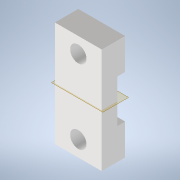
# Autodesk Inventor part: Encoder_Cable_Clamp
Saved by Autodesk Inventor 2022 (Build 260153000, 153)
## iProperties
Created: 2024-05-02
Part Number: Encoder_Cable_Clamp
Material: Generic
Document SubType Name: Modeling
Designer: Gotham City
Density: 1 g/cm^3
Appearance: Default
Author: Gotham City
Autodesk Inventor part; units mm, degrees
ref_plane "YZ Plane" through (0, 0, 0) normal (1, 0, 0) x (0, 1, 0)
ref_plane "XZ Plane" through (0, 0, 0) normal (0, 1, 0) x (-1, 0, 0)
ref_plane "XY Plane" through (0, 0, 0) normal (0, 0, 1) x (1, 0, 0)
sketch "Sketch1" plane through (0, 0, 0) normal (1, 0, 0) x (0, 1, 0)
  line L0 (-0.5, 0) -> (0.55, 0) projected
  line L1 (3.0679, 1.692) -> (-10.4321, 1.692)
  line L2 (-10.4321, 1.692) -> (-10.4321, 4.692)
  line L3 (-10.4321, 4.692) -> (3.0679, 4.692)
  line L4 (3.0679, 4.692) -> (3.0679, 1.692)
  line L5 (-0.9321, 1.692) -> (-6.4321, 1.692)
  line L6 (-6.4321, 1.692) -> (-6.4321, 2.692)
  line L7 (-6.4321, 2.692) -> (-0.9321, 2.692)
  line L8 (-0.9321, 2.692) -> (-0.9321, 1.692)
  line L9 (-3.6821, 1.692) -> (-3.6821, 4.692) construction
  line L10 (1.0679, 4.692) -> (1.0679, 1.692) construction
  line L11 (-0.5, 0) -> (0.55, 0) construction
  point P0 (0, 0)
  dimension "d0" = 5.5
  dimension "d1" = 4
  dimension "d2" = 2
  dimension "d3" = 1
  dimension "d4" = 2
  constraints: 20 end point, 4 parallel, 4 perpendicular, 3 point on line, 2 horizontal, 2 midpoint, 1 other
  measures "d0" distance of L6.end L7.end
  measures "d1" distance between parallel lines of L4 L8
  measures "d2" distance between parallel lines of L3 L7
  measures "d3" distance between parallel lines of L1 L7
  measures "d4" distance between parallel lines of L8 L10
extrude "Extrusion1" add sketch "Sketch1" along normal blind 6 contours L1 L8 L7 L6 L2 L3 L4
sketch "Sketch2" plane through (0, -10.4321, 4.692) normal (0, 0, 1) x (1, 0, 0)
  line L0 (0, 11.5) -> (6, 11.5) construction
  line L1 (6, 13.5) -> (6, 0) construction
  point P0 (0, 10.4321)
  point P1 (3, 11.5)
  constraints: 2 end point, 1 horizontal, 1 midpoint, 1 point on line
hole "Hole1" at (3, 1.0679, 4.692) direction (0, 0, -1) diameter 2.1 end through all clearance for "Socket Head Cap Screw ISO 4762" size "M2" standard "ISO"
ref_plane "Work Plane1" through (0, -3.6821, 4.692) normal (0, 1, 0) x (1, 0, 0)
mirror "Mirror1" about plane through (0, -3.6821, 4.692) normal (0, 1, 0) of "Hole1"
body "Solid1"
